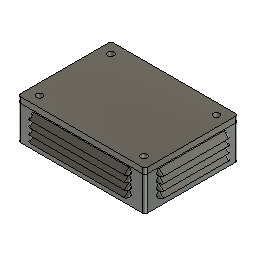
stevenson_box_v1 (Autodesk Fusion 360 design; units mm, degrees)
Autodesk Fusion 360 part; units mm, degrees
note: some values were not read from the file. Chosen so that the rebuilt part matches the saved one: a direction; which bodies a step acts on; which pieces of a blend or face edit are solid. Set by a fixed rule: which sketch regions a step uses.
sketch "Sketch1" plane through (0, 0, 0) normal (0, 0, 1) x (1, 0, 0)
  line L0 (0, 0) -> (100, 0)
  line L1 (100, 0) -> (100, 70)
  line L2 (100, 70) -> (0, 70)
  line L3 (0, 70) -> (0, 0)
  dimension "d4" = 100
  dimension "d5" = 70
  constraint horizontal L0
  constraint vertical L1
  constraint horizontal L2
  constraint vertical L3
  constraint coincident L0.start L3.end
  measures "d4" distance of L0.start L0.end
  measures "d5" distance of L0.start L2.end
extrude "Extrude1" add sketch "Sketch1" along normal blind 6 makes body 1
sketch "Sketch2" plane through (0, 0, 0) normal (0, -1, 0) x (1, 0, 0)
  line L0 (0, 0) -> (100, 0)
  line L1 (100, 0) -> (100, 6)
  line L2 (100, 6) -> (0, 6)
  line L3 (0, 6) -> (0, 0)
  line L4 (0, 0) -> (100, 0)
  line L5 (100, 0) -> (100, 30)
  line L6 (100, 30) -> (0, 30)
  line L7 (0, 30) -> (0, 0)
  dimension "d9" = 100
  dimension "d10" = 30
  constraint horizontal L4
  constraint vertical L5
  constraint horizontal L6
  constraint vertical L7
  constraint coincident L0.start L3.end
  measures "d9" distance of L0.start L0.end
  measures "d10" distance of L0.start L6.end
extrude "Extrude2" add sketch "Sketch2" along normal blind 6 separate body makes body 2
ref_plane "WorkPlane1" through (50, -3, 15) normal (1, 0, 0) x (0, 0, 1)
sketch "Sketch3" plane through (50, 0, 0) normal (1, 0, 0) x (0, 1, 0)
  line L0 (-6, 29) -> (-6, 25)
  line L1 (-6, 25) -> (-10, 25)
  line L2 (-10, 25) -> (-6, 29)
  line L3 (0, 30) -> (-6, 30)
  point P0 (-6, 30)
  point P1 (-6, 0)
  dimension "d15" = 4
  dimension "d16" = 4
  dimension "d87" = 5
  constraint perpendicular L0 L1
  constraint coincident L0 P1
  measures "d15" distance of L0.start L0.end
  measures "d16" distance of L0.end L1.end
  measures "d87" distance of L1 L3
extrude "Extrude3" add sketch "Sketch3" along normal mid plane 87.5 bodies 1 2
fillet "Fillet1" radius 2 2 edges at (6.25, -8, 27) (93.75, -8, 27) on bodies 2
pattern_path "PathPattern1" count 4 spacing 5.75 from (100, -6, 27) backwards along 1 edges at (100, -6, 15) of "Extrude3", "Fillet1" on bodies 2
shell "Shell1" thickness 1 removed faces 4 at (63.9167, -7.3333, 25) at (63.9167, -7.3333, 19.25) at (36.0833, -7.3333, 13.5) at (36.0833, -7.3333, 7.75) on bodies 2
sketch "Sketch4" plane through (0, -1, 0) normal (0, -1, 0) x (1, 0, 0)
  line L0 (99, 1) -> (99, 29)
  line L1 (99, 29) -> (1, 29)
  line L2 (1, 29) -> (1, 1)
  line L3 (91.75, 7.75) -> (91.75, 11.75)
  line L4 (8.25, 11.75) -> (8.25, 7.75)
  line L5 (8.25, 7.75) -> (91.75, 7.75)
  line L6 (93.75, 7.75) -> (91.75, 7.75)
  line L7 (93.75, 7.75) -> (93.75, 8.9216)
  line L8 (91.75, 11.75) -> (91.75, 7.75)
  line L9 (8.25, 7.75) -> (6.25, 7.75)
  line L10 (8.25, 7.75) -> (8.25, 11.75)
  line L11 (6.25, 8.9216) -> (6.25, 7.75)
  line L12 (8.25, 13.5) -> (6.25, 13.5)
  line L13 (8.25, 13.5) -> (8.25, 17.5)
  line L14 (6.25, 14.6716) -> (6.25, 13.5)
  line L15 (91.75, 13.5) -> (91.75, 17.5)
  line L16 (8.25, 17.5) -> (8.25, 13.5)
  line L17 (8.25, 13.5) -> (91.75, 13.5)
  line L18 (93.75, 13.5) -> (91.75, 13.5)
  line L19 (93.75, 13.5) -> (93.75, 14.6716)
  line L20 (91.75, 17.5) -> (91.75, 13.5)
  line L21 (93.75, 19.25) -> (91.75, 19.25)
  line L22 (93.75, 19.25) -> (93.75, 20.4216)
  line L23 (91.75, 23.25) -> (91.75, 19.25)
  line L24 (91.75, 19.25) -> (91.75, 23.25)
  line L25 (8.25, 23.25) -> (8.25, 19.25)
  line L26 (8.25, 19.25) -> (91.75, 19.25)
  line L27 (93.75, 25) -> (91.75, 25)
  line L28 (93.75, 25) -> (93.75, 26.1716)
  line L29 (91.75, 29) -> (91.75, 25)
  line L30 (91.75, 25) -> (91.75, 29)
  line L31 (8.25, 29) -> (8.25, 25)
  line L32 (8.25, 25) -> (91.75, 25)
  line L33 (8.25, 25) -> (6.25, 25)
  line L34 (8.25, 25) -> (8.25, 29)
  line L35 (6.25, 26.1716) -> (6.25, 25)
  line L36 (8.25, 19.25) -> (6.25, 19.25)
  line L37 (8.25, 19.25) -> (8.25, 23.25)
  line L38 (6.25, 20.4216) -> (6.25, 19.25)
  line L39 (1, 1) -> (99, 1)
  ellipse E0 centre (91.75, 8.9216) end of major axis (91.75, 11.75) minor radius 2 (93.75, 8.9216) -> (91.75, 11.75) ccw
  ellipse E1 centre (8.25, 8.9216) end of major axis (8.25, 11.75) minor radius 2 (8.25, 11.75) -> (6.25, 8.9216) ccw
  ellipse E2 centre (8.25, 14.6716) end of major axis (8.25, 17.5) minor radius 2 (8.25, 17.5) -> (6.25, 14.6716) ccw
  ellipse E3 centre (91.75, 14.6716) end of major axis (91.75, 17.5) minor radius 2 (93.75, 14.6716) -> (91.75, 17.5) ccw
  ellipse E4 centre (91.75, 20.4216) end of major axis (91.75, 23.25) minor radius 2 (93.75, 20.4216) -> (91.75, 23.25) ccw
  ellipse E5 centre (91.75, 26.1716) end of major axis (91.75, 29) minor radius 2 (93.75, 26.1716) -> (91.75, 29) ccw
  line L40 (91.75, 29) -> (8.25, 29)
  ellipse E6 centre (8.25, 26.1716) end of major axis (8.25, 29) minor radius 2 (8.25, 29) -> (6.25, 26.1716) ccw
  ellipse E7 centre (8.25, 20.4216) end of major axis (8.25, 23.25) minor radius 2 (8.25, 23.25) -> (6.25, 20.4216) ccw
  line L41 (91.75, 11.75) -> (8.25, 11.75)
  line L42 (91.75, 17.5) -> (8.25, 17.5)
  line L43 (91.75, 23.25) -> (8.25, 23.25)
extrude "Extrude4" cut sketch "Sketch4" against normal blind 6 contours L1 L29 L30 L31 L32 L34 L40 | L3 L4 L5 L8 L10 L41 | L13 L15 L16 L17 L20 L42 | L23 L24 L25 L26 L37 L43 bodies 2
ref_plane "WorkPlane2" through (50, 35, 3) normal (0, 1, 0) x (-1, 0, 0)
mirror "Mirror1" about plane through (50, 35, 3) normal (0, 1, 0) of bodies 2 makes body 4
sketch "Sketch5" plane through (100, 0, 0) normal (1, 0, 0) x (0, 1, 0)
  line L0 (0, 0) -> (70, 0)
  line L1 (70, 0) -> (70, 6)
  line L2 (70, 6) -> (0, 6)
  line L3 (0, 6) -> (0, 0)
  line L4 (-6, 0) -> (76, 0)
  line L5 (76, 0) -> (76, 30)
  line L6 (76, 30) -> (-6, 30)
  line L7 (-6, 30) -> (-6, 0)
  dimension "d29" = 82
  dimension "d30" = 30
  constraint horizontal L4
  constraint vertical L5
  constraint horizontal L6
  constraint vertical L7
  measures "d29" distance of L4.start L4.end
  measures "d30" distance of L4.start L6.end
extrude "Extrude5" add sketch "Sketch5" along normal blind 6 separate body makes body 5
sketch "Sketch6" plane through (0, 0, 6) normal (0, 0, 1) x (-1, 0, 0)
  line L0 (0, -70) -> (0, 0)
  line L1 (0, 0) -> (-100, 0)
  line L2 (-100, 0) -> (-100, -70)
  line L3 (-100, -70) -> (0, -70)
  line L4 (-90, -75.2763) -> (-10, -75.2763)
  line L5 (-10, -75.2763) -> (-10, -25.2763)
  line L6 (-10, -25.2763) -> (-90, -25.2763)
  line L7 (-90, -25.2763) -> (-90, -75.2763)
  line L8 (-90, -75.2763) -> (-10, -25.2763) construction
  line L9 (-10, -75.2763) -> (-90, -25.2763) construction
  line L10 (-10, -75.2763) -> (-15, -75.2763)
  line L11 (-15, -75.2763) -> (-15, -70.2763)
  line L12 (-15, -70.2763) -> (-10, -70.2763)
  line L13 (-10, -70.2763) -> (-10, -75.2763)
  line L14 (-10, -25.2763) -> (-15, -25.2763)
  line L15 (-15, -25.2763) -> (-15, -30.2763)
  line L16 (-15, -30.2763) -> (-10, -30.2763)
  line L17 (-10, -30.2763) -> (-10, -25.2763)
  line L18 (-90, -25.2763) -> (-85, -25.2763)
  line L19 (-85, -25.2763) -> (-85, -30.2763)
  line L20 (-85, -30.2763) -> (-90, -30.2763)
  line L21 (-90, -30.2763) -> (-90, -25.2763)
  line L22 (-90, -75.2763) -> (-85, -75.2763)
  line L23 (-85, -75.2763) -> (-85, -70.2763)
  line L24 (-85, -70.2763) -> (-90, -70.2763)
  line L25 (-90, -70.2763) -> (-90, -75.2763)
  point P0 (-50, -50.2763)
  dimension "d33" = 80
  dimension "d34" = 50
  dimension "d40" = 5
  dimension "d45" = 5
  dimension "d46" = 5
  dimension "d49" = 10
  dimension "d50" = 5
  dimension "d51" = 5
  dimension "d52" = 5
  dimension "d53" = 5
  dimension "d54" = 5
  constraint horizontal L4
  constraint perpendicular L4 L5
  constraint parallel L4 L6
  constraint parallel L5 L7
  constraint coincident L8 P0
  constraint coincident L9 P0
  constraint horizontal L10
  constraint vertical L11
  constraint horizontal L12
  constraint vertical L13
  constraint horizontal L14
  constraint vertical L15
  constraint horizontal L16
  constraint vertical L17
  constraint horizontal L18
  constraint vertical L19
  constraint horizontal L20
  constraint vertical L21
  constraint horizontal L22
  constraint vertical L23
  constraint horizontal L24
  constraint vertical L25
  measures "d33" distance of L5.end L6.end
  measures "d34" distance of L4.end L5.end
  measures "d40" distance of L10.end L11.end
  measures "d45" distance of L22.end L23.end
  measures "d46" distance of L18.end L19.end
  measures "d49" distance of L2 L7
  measures "d50" distance of L14.end L15.end
  measures "d51" distance of L15.end L16.end
  measures "d52" distance of L11.end L12.end
  measures "d53" distance of L23.end L24.end
  measures "d54" distance of L19.end L20.end
ref_plane "WorkPlane3" through (103, 35, 15) normal (0, 1, 0) x (0, 0, 1)
sketch "Sketch7" plane through (0, 35, 0) normal (0, 1, 0) x (1, 0, 0)
  line L0 (106, -29) -> (106, -25)
  line L1 (106, -25) -> (110, -25)
  line L2 (110, -25) -> (106, -29)
  point P0 (106, -30)
  dimension "d55" = 4
  dimension "d56" = 4
  dimension "d88" = 5
  constraint vertical L0
  constraint perpendicular L0 L1
  constraint coincident L0 P0
  measures "d55" distance of L0.start L0.end
  measures "d56" distance of L0.end L1.end
  measures "d88" distance of L1 P0
extrude "Extrude8" add sketch "Sketch7" along normal mid plane 61.25 bodies 5
fillet "Fillet2" radius 2 2 edges at (108, 4.375, 27) (108, 65.625, 27) on bodies 5
pattern_path "PathPattern2" count 4 spacing 5.65 from (106, -6, 26.7) along 1 edges at (106, -6, 15) of "Extrude8", "Fillet2" on bodies 5
ref_plane "WorkPlane4" through (50, 35, 3) normal (-1, 0, 0) x (0, -1, 0)
shell "Shell2" thickness 1 removed faces 4 at (107.3333, 44.5417, 25) at (107.3333, 44.5417, 19.35) at (107.3333, 44.5417, 13.7) at (107.3333, 25.4583, 8.05) on bodies 5
sketch "Sketch9" plane through (106, 0, 0) normal (1, 0, 0) x (0, 1, 0)
  line L0 (-6, 30) -> (-6, 0)
  line L1 (-6, 0) -> (76, 0)
  line L2 (76, 0) -> (76, 30)
  line L3 (76, 30) -> (-6, 30)
  line L4 (63.625, 25) -> (63.625, 29)
  line L5 (6.375, 29) -> (6.375, 25)
  line L6 (6.375, 25) -> (63.625, 25)
  line L7 (63.625, 19.35) -> (63.625, 23.35)
  line L8 (6.375, 23.35) -> (6.375, 19.35)
  line L9 (6.375, 19.35) -> (63.625, 19.35)
  line L10 (63.625, 13.7) -> (63.625, 17.7)
  line L11 (6.375, 17.7) -> (6.375, 13.7)
  line L12 (6.375, 13.7) -> (63.625, 13.7)
  line L13 (63.625, 8.05) -> (63.625, 12.05)
  line L14 (6.375, 12.05) -> (6.375, 8.05)
  line L15 (6.375, 8.05) -> (63.625, 8.05)
  line L16 (65.625, 9.2216) -> (65.625, 8.05)
  line L17 (4.375, 8.05) -> (4.375, 9.2216)
  line L18 (65.625, 8.05) -> (64.625, 8.05)
  ellipse E0 centre (6.375, 9.2216) end of major axis (6.375, 12.05) minor radius 2 (6.375, 12.05) -> (4.375, 9.2216) ccw
  line L19 (65.625, 13.7) -> (64.625, 13.7)
  ellipse E1 centre (6.375, 14.8716) end of major axis (6.375, 17.7) minor radius 2 (6.375, 17.7) -> (4.375, 14.8716) ccw
  line L20 (65.625, 19.35) -> (64.625, 19.35)
  ellipse E2 centre (6.375, 20.5216) end of major axis (6.375, 23.35) minor radius 2 (6.375, 23.35) -> (4.375, 20.5216) ccw
  line L21 (64.625, 25) -> (5.375, 25)
  line L22 (4.375, 25) -> (4.375, 26.1716)
  ellipse E3 centre (6.375, 26.1716) end of major axis (6.375, 29) minor radius 2 (6.375, 29) -> (4.375, 26.1716) ccw
  line L23 (6.375, 29) -> (63.625, 29)
  ellipse E4 centre (63.625, 26.1716) end of major axis (63.625, 29) minor radius 2 (65.625, 26.1716) -> (63.625, 29) ccw
  line L24 (65.625, 25) -> (64.625, 25)
  ellipse E5 centre (63.625, 20.5216) end of major axis (63.625, 23.35) minor radius 2 (65.625, 20.5216) -> (63.625, 23.35) ccw
  ellipse E6 centre (63.625, 14.8716) end of major axis (63.625, 17.7) minor radius 2 (65.625, 14.8716) -> (63.625, 17.7) ccw
  ellipse E7 centre (63.625, 9.2216) end of major axis (63.625, 12.05) minor radius 2 (65.625, 9.2216) -> (63.625, 12.05) ccw
  line L25 (63.625, 29) -> (6.375, 29)
  line L26 (6.375, 12.05) -> (63.625, 12.05)
  line L27 (64.625, 8.05) -> (5.375, 8.05)
  line L28 (5.375, 8.05) -> (4.375, 8.05)
  line L29 (4.375, 13.7) -> (4.375, 14.8716)
  line L30 (6.375, 17.7) -> (63.625, 17.7)
  line L31 (65.625, 14.8716) -> (65.625, 13.7)
  line L32 (64.625, 13.7) -> (5.375, 13.7)
  line L33 (5.375, 13.7) -> (4.375, 13.7)
  line L34 (4.375, 19.35) -> (4.375, 20.5216)
  line L35 (6.375, 23.35) -> (63.625, 23.35)
  line L36 (65.625, 20.5216) -> (65.625, 19.35)
  line L37 (64.625, 19.35) -> (5.375, 19.35)
  line L38 (5.375, 19.35) -> (4.375, 19.35)
  line L39 (65.625, 26.1716) -> (65.625, 25)
  line L40 (5.375, 25) -> (4.375, 25)
  line L41 (63.625, 23.35) -> (6.375, 23.35)
  line L42 (63.625, 17.7) -> (6.375, 17.7)
  line L43 (63.625, 12.05) -> (6.375, 12.05)
extrude "Extrude9" cut sketch "Sketch9" against normal blind 6 contours L4 L5 L6 L21 L23 L25 | L7 L8 L9 L35 L37 L41 | L10 L11 L12 L30 L32 L42 | L13 L14 L15 L26 L27 L43 bodies 5
mirror "Mirror3" about plane through (50, 35, 3) normal (-1, 0, 0) of bodies 5 makes body 6
combine "Combine1" operation add target body 6 tool bodies 2 5 4 1
fillet "Fillet3" radius 2 4 edges at (106, 76, 15) (106, -6, 15) (-6, 76, 15) (-6, -6, 15) on bodies 6
sketch "Sketch10" plane through (0, 0, 30) normal (0, 0, 1) x (-1, 0, 0)
  line L0 (4, 6) -> (-104, 6)
  arc A0 (-104, 6) -> (-106, 4) centre (-104, 4) ccw
  line L1 (-106, 4) -> (-106, -74)
  arc A1 (-106, -74) -> (-104, -76) centre (-104, -74) ccw
  line L2 (-104, -76) -> (4, -76)
  line L3 (-100, 0) -> (0, 0)
  circle A2 centre (0, 0) radius 10
  circle A3 centre (-100, -70) radius 10
  circle A4 centre (0, -70) radius 10
  circle A5 centre (-100, 0) radius 10
  line L4 (0, -70) -> (-100, -70)
  line L5 (6, -74) -> (6, 4)
  arc A6 (6, 4) -> (4, 6) centre (4, 4) ccw
  arc A7 (4, -76) -> (6, -74) centre (4, -74) ccw
  line L6 (-100, -70) -> (-100, 0)
  line L7 (0, 0) -> (0, -70)
  dimension "d90" = 20
  dimension "d91" = 20
  dimension "d92" = 20
  dimension "d93" = 20
  constraint coincident A4.centre L4.start
  constraint coincident L3.start A5.centre
  constraint coincident A3.centre L4.end
  constraint coincident L3.end A2.centre
  measures "d90" diameter of A5
  measures "d91" diameter of A3
  measures "d92" diameter of A4
  measures "d93" diameter of A2
extrude "Extrude10" add sketch "Sketch10" against normal blind 10 separate body contours L3 A2 L7 | L3 A5 L6 | A4 L4 L7 | A3 L4 L6 makes body 7 at (90.0113, 0.4758, 23.3333) makes body 8 at (9.9887, 0.4758, 26.6667) makes body 9 at (90.7163, 66.2834, 23.3333) makes body 10 at (8.8884, 65.4177, 23.3333)
combine "Combine2" operation add target body 9 tool bodies 6 7 8
sketch "Sketch11" plane through (0, 0, 30) normal (0, 0, 1) x (-1, 0, 0)
  arc A0 (6, 4) -> (4, 6) centre (4, 4) ccw
  line L0 (4, 6) -> (-104, 6)
  arc A1 (-104, 6) -> (-106, 4) centre (-104, 4) ccw
  line L1 (-106, 4) -> (-106, -74)
  arc A2 (-106, -74) -> (-104, -76) centre (-104, -74) ccw
  line L2 (-104, -76) -> (4, -76)
  arc A3 (4, -76) -> (6, -74) centre (4, -74) ccw
  line L3 (6, -74) -> (6, 4)
  arc A4 (-90, -70) -> (-100, -60) centre (-100, -70) ccw
  line L4 (-100, -60) -> (-100, -10)
  arc A5 (-100, -10) -> (-90, 0) centre (-100, 0) ccw
  line L5 (-90, 0) -> (-10, 0)
  arc A6 (-10, 0) -> (0, -10) centre (0, 0) ccw
  line L6 (0, -10) -> (0, -70)
  line L7 (0, -70) -> (-90, -70)
  circle A7 centre (-3.5355, -66.4645) radius 1.2674
  circle A8 centre (-3.9043, -3.1235) radius 2
  circle A9 centre (-96.4645, -66.4645) radius 3
  circle A10 centre (-96, -3) radius 1
  dimension "d94" = 5
  dimension "d95" = 5
  dimension "d96" = 5
  dimension "d97" = 5
  measures "d94" distance of L6.end A7.centre
  measures "d95" distance of A4.centre A9.centre
  measures "d96" distance of A5.centre A10.centre
  measures "d97" distance of A6.centre A8.centre
hole "Hole1" at (3.9043, 3.1235, 30) at (96.4645, 66.4645, 30) at (96, 3, 30) at (3.5355, 66.4645, 30) direction (0, 0, -1) diameter 5.4 depth 15 tip angle 118 bodies 10 9
sketch "Sketch12" plane through (0, 0, 30) normal (0, 0, 1) x (-1, 0, 0)
  arc A0 (-90, -70) -> (-100, -60) centre (-100, -70) ccw
  line L0 (-100, -60) -> (-100, -10)
  arc A1 (-100, -10) -> (-90, 0) centre (-100, 0) ccw
  line L1 (-90, 0) -> (-10, 0)
  arc A2 (-10, 0) -> (0, -10) centre (0, 0) ccw
  line L2 (0, -10) -> (0, -70)
  line L3 (0, -70) -> (-90, -70)
  arc A3 (-104, 6) -> (-106, 4) centre (-104, 4) ccw
  line L4 (-106, 4) -> (-106, -74)
  arc A4 (-106, -74) -> (-104, -76) centre (-104, -74) ccw
  line L5 (-104, -76) -> (4, -76)
  arc A5 (4, -76) -> (6, -74) centre (4, -74) ccw
  line L6 (6, -74) -> (6, 4)
  arc A6 (6, 4) -> (4, 6) centre (4, 4) ccw
  line L7 (4, 6) -> (-104, 6)
  circle A7 centre (-96.4645, -66.4645) radius 2.7
  circle A8 centre (-3.9043, -3.1235) radius 2.7
  circle A9 centre (-96, -3) radius 2.7
  circle A10 centre (-3.5355, -66.4645) radius 1.2674
  arc A11 (0, -60) -> (-10, -70) centre (0, -70) ccw
  circle A12 centre (-3.5355, -66.4645) radius 2.7
  arc A13 (0, -60) -> (-10, -70) centre (0, -70) ccw
  dimension "d98" = 5.4
  constraint concentric A10 A12
  constraint concentric A11 A13
  measures "d98" diameter of A12
extrude "Extrude11" add sketch "Sketch12" along normal blind 5 separate body contours A0 L0 A1 L1 A2 L2 L3 A11 A13 | L2 L3 A11 A13 | A3 L4 A4 L5 A5 L6 A6 L7 makes body 11
combine "Combine4" operation add target body 10 tool bodies 9
sketch "Sketch13" plane through (106, 0, 0) normal (1, 0, 0) x (0, 1, 0)
  line L0 (4.375, 8.05) -> (4.375, 9.2216)
  ellipse E0 centre (6.375, 9.2216) end of major axis (6.375, 12.05) minor radius 2 (6.375, 12.05) -> (4.375, 9.2216) ccw
  line L1 (6.375, 12.05) -> (63.625, 12.05)
  ellipse E1 centre (63.625, 9.2216) end of major axis (63.625, 12.05) minor radius 2 (65.625, 9.2216) -> (63.625, 12.05) ccw
  line L2 (65.625, 9.2216) -> (65.625, 8.05)
  line L3 (65.625, 8.05) -> (64.625, 8.05)
  line L4 (64.625, 8.05) -> (5.375, 8.05)
  line L5 (5.375, 8.05) -> (4.375, 8.05)
  line L6 (4.375, 13.7) -> (4.375, 14.8716)
  ellipse E2 centre (6.375, 14.8716) end of major axis (6.375, 17.7) minor radius 2 (6.375, 17.7) -> (4.375, 14.8716) ccw
  line L7 (6.375, 17.7) -> (63.625, 17.7)
  ellipse E3 centre (63.625, 14.8716) end of major axis (63.625, 17.7) minor radius 2 (65.625, 14.8716) -> (63.625, 17.7) ccw
  line L8 (65.625, 14.8716) -> (65.625, 13.7)
  line L9 (65.625, 13.7) -> (64.625, 13.7)
  line L10 (64.625, 13.7) -> (5.375, 13.7)
  line L11 (5.375, 13.7) -> (4.375, 13.7)
  line L12 (4.375, 19.35) -> (4.375, 20.5216)
  ellipse E4 centre (6.375, 20.5216) end of major axis (6.375, 23.35) minor radius 2 (6.375, 23.35) -> (4.375, 20.5216) ccw
  line L13 (6.375, 23.35) -> (63.625, 23.35)
  ellipse E5 centre (63.625, 20.5216) end of major axis (63.625, 23.35) minor radius 2 (65.625, 20.5216) -> (63.625, 23.35) ccw
  line L14 (65.625, 20.5216) -> (65.625, 19.35)
  line L15 (65.625, 19.35) -> (64.625, 19.35)
  line L16 (64.625, 19.35) -> (5.375, 19.35)
  line L17 (5.375, 19.35) -> (4.375, 19.35)
  line L18 (4.375, 25) -> (4.375, 26.1716)
  ellipse E6 centre (6.375, 26.1716) end of major axis (6.375, 29) minor radius 2 (6.375, 29) -> (4.375, 26.1716) ccw
  line L19 (6.375, 29) -> (63.625, 29)
  ellipse E7 centre (63.625, 26.1716) end of major axis (63.625, 29) minor radius 2 (65.625, 26.1716) -> (63.625, 29) ccw
  line L20 (65.625, 26.1716) -> (65.625, 25)
  line L21 (65.625, 25) -> (64.625, 25)
  line L22 (64.625, 25) -> (5.375, 25)
  line L23 (5.375, 25) -> (4.375, 25)
  line L24 (-4, 30) -> (-4, 0)
  line L25 (-4, 0) -> (74, 0)
  line L26 (74, 0) -> (74, 30)
  line L27 (74, 30) -> (-4, 30)
equation "box_length = 100 mm"
equation "box_width = 70 mm"
equation "box_height = 30 mm"
equation "d4 = box_length"
equation "d5 = box_width"
equation "box_thickness = 6 mm"
equation "d7 = box_thickness"
equation "d9 = box_length"
equation "d10 = box_height"
equation "d11 = box_thickness"
equation "vent_length = 4 mm"
equation "d15 = vent_length"
equation "d16 = vent_length"
equation "d17 = ( box_length / 2 ) * 7 / 8"
equation "vent_fillet = 2 mm"
equation "d21 = vent_fillet"
equation "d23 = box_height * 7 / 8 - box_thickness"
equation "d25 = -box_thickness"
equation "d29 = box_width + 2 * box_thickness"
equation "d30 = box_height"
equation "d31 = box_thickness"
equation "d33 = breadboard_length"
equation "d34 = breadboard_width"
equation "d40 = center_stands"
equation "center_stands = 5 mm"
equation "breadboard_length = 80 mm"
equation "breadboard_width = 50 mm"
equation "d45 = center_stands"
equation "d46 = center_stands"
equation "d49 = ( box_length - breadboard_length ) / 2"
equation "d50 = center_stands"
equation "d51 = center_stands"
equation "d52 = center_stands"
equation "d53 = center_stands"
equation "d54 = center_stands"
equation "d55 = vent_length"
equation "d56 = vent_length"
equation "d57 = box_width / 2 * 7 / 8"
equation "d60 = vent_fillet"
equation "d62 = box_height * 7 / 8 - box_thickness"
equation "d66 = -box_thickness"
equation "d71 = vent_fillet"
equation "d87 = box_height / 6"
equation "d88 = box_height / 6"
equation "top_circle = 20 mm"
equation "d90 = top_circle"
equation "d91 = top_circle"
equation "d92 = top_circle"
equation "d93 = top_circle"
equation "d94 = top_circle / 4"
equation "d95 = top_circle / 4"
equation "d96 = top_circle / 4"
equation "d97 = top_circle / 4"
named bodies: "stevensonLid", "stevensonBody"
